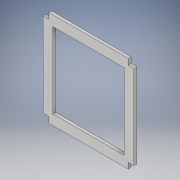
# Autodesk Inventor part: Upper Platform
Saved by Autodesk Inventor 2018 (Build 220112000, 112)
## iProperties
Created: 2019-01-10
Part Number: Upper Platform
Material: Generic
Document SubType Name: Modeling
Designer: maste
Density: 1 g/cm^3
Appearance: Default
Author: maste
Autodesk Inventor part; units mm, degrees
ref_plane "YZ Plane" through (0, 0, 0) normal (1, 0, 0) x (0, 1, 0)
ref_plane "XZ Plane" through (0, 0, 0) normal (0, 1, 0) x (-1, 0, 0)
ref_plane "XY Plane" through (0, 0, 0) normal (0, 0, 1) x (1, 0, 0)
sketch "Sketch1" plane through (0, 0, 0) normal (0, 0, 1) x (1, 0, 0)
  line L0 (0, 0) -> (692.4548, 0)
  line L1 (692.4548, 0) -> (692.4548, 50.8)
  line L2 (692.4548, 50.8) -> (743.2548, 50.8)
  line L3 (743.2548, 50.8) -> (743.2548, 787.4)
  line L4 (743.2548, 787.4) -> (692.4548, 787.4)
  line L5 (692.4548, 787.4) -> (692.4548, 838.2)
  line L6 (692.4548, 838.2) -> (0, 838.2)
  line L7 (0, 838.2) -> (0, 787.4)
  line L8 (0, 787.4) -> (-50.8, 787.4)
  line L9 (-50.8, 787.4) -> (-50.8, 50.8)
  line L10 (-50.8, 50.8) -> (0, 50.8)
  line L11 (0, 50.8) -> (0, 0)
  line L12 (692.4548, 787.4) -> (0, 50.8) construction
  line L13 (692.4548, 50.8) -> (0, 787.4) construction
  line L14 (692.4548, 787.4) -> (657.66, 750.387) construction
  line L15 (657.66, 750.387) -> (34.7948, 750.387)
  line L16 (34.7948, 750.387) -> (34.7948, 87.813)
  line L17 (34.7948, 87.813) -> (657.66, 87.813)
  line L18 (657.66, 87.813) -> (657.66, 750.387)
  dimension "d0" = 692.4548
  dimension "d1" = 50.8
  dimension "d2" = 50.8
  dimension "d3" = 736.6
  dimension "d4" = 50.8
  dimension "d5" = 50.8
  dimension "d6" = 50.8
  dimension "d7" = 50.8
  constraints: 38 end point, 11 point on line, 9 perpendicular, 2 horizontal
  measures "d0" distance of L0.start L0.end
  measures "d1" distance of L0.end L1.end
  measures "d2" distance of L1.end L2.end
  measures "d3" distance of L2.end L3.end
  measures "d4" distance of L4.end L5.end
  measures "d5" distance of L6.end L7.end
  measures "d6" distance of L7.end L8.end
  measures "d7" distance of L4.end L14.end
extrude "Extrusion1" add sketch "Sketch1" along normal blind 25.4
body "Solid1"
